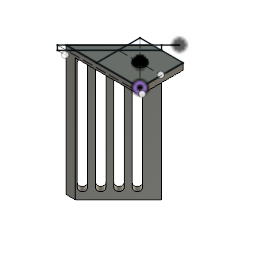
HOLDER_ESP32_S3_CAM (Autodesk Fusion 360 design; units mm, degrees)
part number: 2025-12-13-19-33-31-146
Autodesk Fusion 360 part; units mm, degrees
sketch "Sketch1" plane through (0, 0, 0) normal (0, 0, 1) x (1, 0, 0)
  line L0 (0, 0) -> (-20, 0)
  line L1 (-20, 0) -> (-20, 20)
  line L2 (-20, 20) -> (0, 20)
  line L3 (0, 20) -> (0, 0)
  line L4 (-20, 20) -> (0, 0) construction
  circle A0 centre (-10, 10) radius 2.6
  line L5 (-10, 20) -> (-20, 10)
  line L6 (-20, 10) -> (-34.1421, -4.1421)
  line L7 (-20, 10) -> (-0.3454, 10) construction
  line L8 (-34.1421, -4.1421) -> (-36.2635, -2.0208)
  line L9 (-34.1421, -4.1421) -> (-30.4876, -4.1421) construction
  line L10 (-36.2635, -2.0208) -> (-7.9792, 26.2635)
  line L11 (-36.2635, -2.0208) -> (3.0294, -2.0208) construction
  line L12 (-10, 20) -> (-12.1213, 22.1213)
  line L13 (-20, 0) -> (-34.2426, 0)
  dimension "d5" = 20
  dimension "d6" = 20
  dimension "d7" = 5.2
  dimension "d8" = 135
  dimension "d9" = 20
  dimension "d10" = 135
  dimension "d11" = 3
  dimension "d14" = 45
  dimension "d15" = 40
  constraint horizontal L0
  constraint vertical L1
  constraint horizontal L2
  constraint vertical L3
  constraint coincident L0.start L3.end
  constraint midpoint L4 A0.centre
  constraint midpoint L2 L5.start
  constraint midpoint L1 L5.end
  constraint horizontal L7
  constraint horizontal L9
  constraint horizontal L11
  constraint coincident L10 L12.end
  constraint perpendicular L10 L12
  constraint coincident L10 L13.end
  constraint perpendicular L1 L13
  measures "d5" distance of L0.start L0.end
  measures "d6" distance of L0.start L2.end
  measures "d7" diameter of A0
  measures "d8" angle of L6 L7
  measures "d9" distance of L5.end L6.end
  measures "d10" angle of L8 L9
  measures "d11" distance of L6.end L8.end
  measures "d14" angle of L10 L11
  measures "d15" distance of L8.end L10.end
extrude "Extrude1" add sketch "Sketch1" against normal blind 3 contours L0 L1 L2 L3 L5 | L1 L6 L13 makes body 1
extrude "Extrude2" add sketch "Sketch1" against normal blind 60 separate body contours L1 L6 L10 L13 | L1 L2 L5 L10 makes body 2
sketch "Sketch2" plane through (-17.1213, 17.1213, 0) normal (-0.707107, 0.707107, 0) x (-0.707107, -0.707107, 0)
  line L0 (24.2132, 0) -> (-4.0711, 0)
  line L1 (-4.0711, 0) -> (-4.0711, -60)
  line L2 (-4.0711, -60) -> (24.2132, -60)
  line L3 (24.2132, -60) -> (24.2132, 0)
  line L4 (24.2132, -30) -> (-4.0711, -30) construction
  line L5 (17.1608, -55) -> (20.5608, -55) construction
  line L6 (20.5608, -55) -> (20.5608, -5)
  line L7 (20.5608, -5) -> (17.1608, -5) construction
  line L8 (17.1608, -5) -> (17.1608, -55)
  line L9 (17.1608, -55) -> (20.5608, -5) construction
  line L10 (20.5608, -55) -> (17.1608, -5) construction
  arc A0 (17.1765, -54.7699) -> (20.5452, -54.7699) centre (18.8608, -55) ccw
  arc A1 (20.5452, -5.2301) -> (17.1765, -5.2301) centre (18.8608, -5) ccw
  arc A2 (11.1765, -54.7699) -> (14.5452, -54.7699) centre (12.8608, -55) ccw
  line L11 (14.5608, -55) -> (14.5608, -5)
  line L12 (11.1608, -5) -> (11.1608, -55)
  arc A3 (14.5452, -5.2301) -> (11.1765, -5.2301) centre (12.8608, -5) ccw
  arc A4 (5.1765, -54.7699) -> (8.5452, -54.7699) centre (6.8608, -55) ccw
  line L13 (8.5608, -55) -> (8.5608, -5)
  line L14 (5.1608, -5) -> (5.1608, -55)
  arc A5 (8.5452, -5.2301) -> (5.1765, -5.2301) centre (6.8608, -5) ccw
  arc A6 (-0.8235, -54.7699) -> (2.5452, -54.7699) centre (0.8608, -55) ccw
  line L15 (2.5608, -55) -> (2.5608, -5)
  line L16 (-0.8392, -5) -> (-0.8392, -55)
  arc A7 (2.5452, -5.2301) -> (-0.8235, -5.2301) centre (0.8608, -5) ccw
  point P0 (18.8608, -30)
  dimension "d23" = 3.4
  dimension "d24" = 50
  dimension "d27" = -6
  dimension "d28" = 0
  constraint midpoint L3 L4.start
  constraint midpoint L1 L4.end
  constraint horizontal L5
  constraint perpendicular L5 L6
  constraint parallel L5 L7
  constraint parallel L6 L8
  constraint coincident L9 P0
  constraint coincident L10 P0
  constraint coincident L4 P0
  constraint midpoint L7 A1.centre
  constraint coincident L7.end A1
  constraint midpoint L5 A0.centre
  constraint coincident L5.start A0
  constraint coincident L10 A0.end
  constraint coincident L9 A0.start
  constraint coincident L10 A1.end
  constraint coincident L9 A1.start
  measures "d23" distance of L6.end L7.end
  measures "d24" distance of L5.end L6.end
extrude "Extrude3" cut sketch "Sketch2" against normal blind 3 contours L6 L8 A0 A1 | A2 L11 L12 A3 | A4 L13 L14 A5 | A6 L15 L16 A7 bodies 2
combine "Combine1" operation add target body 1 tool bodies 2
equation "holder_depth = 20 mm"
equation "holder_width = 20 mm"
equation "d5 = holder_width"
equation "d6 = holder_depth"
equation "d7 = m5_hole"
equation "d11 = holder_base_height"
equation "holder_base_height = 3 mm"
equation "holder_height = 60 mm"
equation "d18 = -holder_base_height"
equation "d20 = -holder_height"
equation "d23 = m3_hole"
equation "d24 = holder_height - 10 mm"
equation "d29 = -holder_base_height"
equation "m3_hole = 3.4 mm"
equation "m5_hole = 5.2 mm"
